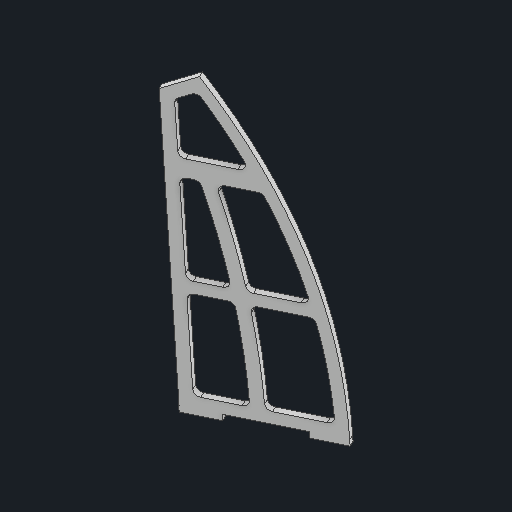
# Autodesk Inventor part: sponson_spanner_bottom
Saved by Autodesk Inventor 2023 (Build 270158030, 158C)
## iProperties
Created: 2022-03-22
Part Number: sponson_spanner_bottom
Material: Generic
Document SubType Name: Modeling
Designer: kardo
Density: 1 g/cm^3
Appearance: Default
Mass: 2.79206 g
Surface Area: 40.129 cm^2
Volume: 2.79206 cm^3
Author: kardo
Autodesk Inventor part; units mm, degrees
ref_plane "YZ Plane" through (0, 0, 0) normal (1, 0, 0) x (0, 1, 0)
ref_plane "XZ Plane" through (0, 0, 0) normal (0, 1, 0) x (-1, 0, 0)
ref_plane "XY Plane" through (0, 0, 0) normal (0, 0, 1) x (1, 0, 0)
derived "parameters_frame.ipt"
derived "stencil_frame.ipt"
sketch "sk_joint_locations" plane through (81.12, 0, 0) normal (1, 0, 0) x (0, 1, 0)
  line L0 (0, 0) -> (111.39, 7.7891) construction
  line L1 (30.81, 28.832) -> (94.8, 28.832) construction
  arc A0 (30.81, 28.832) -> (9.48, 28.5282) centre (30.81, -720.1791) ccw construction
  line L2 (-254.1001, 21.0191) -> (9.48, 28.5282) construction
  line L3 (-363, 18.496) -> (-275.8801, 20.463) construction
  arc A1 (-275.8801, 20.463) -> (-254.1001, 21.0191) centre (-359.1231, 3707.4463) ccw construction
  line L4 (-210.8824, 4616.4994) -> (225.0382, -1617.4555) construction
  line L5 (-242.0001, 4592.9714) -> (-242.0001, -1605.7041) construction
  line L6 (-120.9999, 4592.9714) -> (-120.9999, -1605.7041) construction
  line L7 (-363, 4592.9714) -> (-363, -1605.7041) construction
  line L8 (0, 4592.9714) -> (0, -1605.7041) construction
  line L9 (551.8244, 47.4419) -> (-603.6686, 7.0912) construction
  line L10 (-657.8036, -26.1228) -> (709.4042, 69.4817) construction
  line L11 (178.2183, 30.3929) -> (177.9391, 38.388) construction
  line L12 (185.9231, 36.8959) -> (186.4825, 28.8959) construction
  line L13 (0, 6.528) -> (111.1168, 11.6964) construction
  line L14 (-242.0001, 45.8501) -> (-242.0001, 21.3638) construction
  line L15 (-363, 37.4293) -> (-363, 18.496) construction
  line L16 (-120.9999, 51.0063) -> (-120.9999, 24.811) construction
  line L17 (0, 52.89) -> (0, 28.2581) construction
  line L18 (108.3896, 50.6971) -> (108.935, 42.897) construction
  line L19 (109.4805, 35.0968) -> (108.935, 42.897) construction
  line L20 (109.4805, 35.0968) -> (110.0259, 27.2967) construction
  line L21 (110.0259, 27.2967) -> (110.5713, 19.4965) construction
  line L22 (110.5713, 19.4965) -> (111.1168, 11.6964) construction
  line L23 (0, 6.528) -> (0, 0) construction
  line L24 (94.8, 37.536) -> (94.8, 28.832) construction
  line L25 (94.8, 35.548) -> (94.8, 30.82) construction
  spline S0 degree 4 poles (-363, 37.4293) (-272.3626, 45.1427) (-181.5879, 49.7528) (-90.8131, 52.89) (0, 52.89) knots 0 0 0 0 0 1 1 1 1 1
  spline S1 degree 3 poles (0, 52.89) (86.3106, 52.89) (181.3207, 49.5034) (237, 36.448) knots 0 0 0 0 1 1 1 1
  spline S2 degree 2 poles (111.39, 7.7891) (176.0348, 12.3096) (237, 36.448) knots 0 0 0 1 1 1
  point P0 (-210.8824, 4616.4994)
  point P1 (225.0382, -1617.4555)
  point P2 (178.0787, 34.3904)
  point P3 (186.2028, 32.8959)
  point P4 (134.9575, 11.3411)
  point P5 (-363, 27.9627)
  point P6 (-242.0001, 33.6069)
  point P7 (-120.9999, 37.9086)
  point P8 (0, 40.5741)
  point P9 (94.8, 33.184)
sketch "sk_spanner_joints_locations" plane through (0, 111.39, 7.7891) normal (0, 0.9975641, 0.0697565) x (-1, 0, 0)
  line L0 (270.3063, 10.9615) -> (-449.6313, 38.2305) construction
  line L1 (-853.4143, -320.9901) -> (1860.1762, 876.5297) construction
  line L2 (-85.1788, 24.4262) -> (-84.0523, 18.5329) construction
  line L3 (-85.1788, 24.4262) -> (-71.8427, 23.9211) construction
  line L4 (-84.0523, 18.5329) -> (-71.8427, 23.9211) construction
  point P0 (0, 0)
  point P1 (-126.048, 0)
  point P2 (-156, 27.1087)
  point P3 (-141.8358, 26.5722)
  point P4 (-99.343, 24.9627)
  point P5 (-94.5512, 13.8997)
  point P6 (-115.5491, 4.6332)
ref_plane "plane_strnger_outer" through (84.12, 0, 0) normal (1, 0, 0) x (0, 1, 0)
sketch "sk_corner_offset" plane through (0, 111.39, 7.7891) normal (0, 0.9975641, 0.0697565) x (-1, 0, 0)
  line L0 (-156, 27.1087) -> (-126.048, 0) construction
  line L1 (-126.048, 0) -> (-81.12, 0) construction
  point P0 (0, 0)
  point P1 (-125.5856, 1.2)
  dimension "d7" = 1.2
  dimension "d8" = 1.2
  constraints: 4 end point, 1 horizontal
  measures "d7" distance from line of L0 point (-125.586, 1.2)
  measures "d8" distance from line of point (-125.586, 1.2) L1
sketch "sk_tip_offset" plane through (81.12, 0, 0) normal (1, 0, 0) x (0, 1, 0)
  spline S0 degree 3 poles (0, 52.89) (86.3106, 52.89) (181.3207, 49.5034) (237, 36.448) knots 0 0 0 0 1 1 1 1 construction
  spline S1 degree 2 poles (111.39, 7.7891) (176.0348, 12.3096) (237, 36.448) knots 0 0 0 1 1 1 construction
  spline S2 degree 5 poles (0, 51.69) (13.1181, 51.69) (26.2363, 51.6248) (39.354, 51.4874) (65.3463, 51.0551) (91.3298, 50.254) (104.1978, 49.754) (128.8047, 48.5691) (153.3792, 46.8416) (165.0971, 45.8705) (185.7675, 43.844) (206.3487, 41.0607) (215.2522, 39.6762) (224.1241, 38.0772) (232.9228, 36.143) knots 0 0 0 0 0 0 0.280538 0.280538 0.280538 0.555921 0.555921 0.555921 0.807344 0.807344 0.807344 1 1 1 1 1 1
  spline S3 degree 5 poles (111.3063, 8.9862) (136.261, 10.7315) (161.0871, 14.3225) (185.5959, 19.817) (209.5823, 27.1424) (232.9228, 36.1431) knots 0 0 0 0 0 0 1 1 1 1 1 1
  point P0 (0, 0)
  dimension "d9" = 1.2
  dimension "d10" = 1.2
  constraints: 1 coincident, 6 other
sketch "sk_spanner_bottom_base" plane through (126.048, 0, 0) normal (0.4037383, -0.0638184, 0.9126459) x (-0.1841621, 0.9714748, 0.1494022)
  spline S0 degree 2 poles (109.3763, -22.4773) (178.4423, -36.6707) (243.959, 0) knots 0 0 0 1 1 1 construction
  line L0 (-581.1403, 166.2138) -> (698.1316, -96.6821) projected
  line L1 (109.559, -21.5883) -> (107.5999, -21.1858)
  line L2 (107.5999, -21.1858) -> (109.7273, -10.8338)
  line L3 (109.7273, -10.8338) -> (111.6863, -11.2364)
  line L4 (111.6863, -11.2364) -> (116.3065, 11.2454)
  line L5 (116.3065, 11.2454) -> (114.3474, 11.648)
  line L6 (114.3474, 11.648) -> (116.6574, 22.8889)
  line L7 (116.6574, 22.8889) -> (118.6165, 22.4863)
  line L8 (118.6165, 22.4863) -> (118.6016, 22.4138)
  line L9 (109.3763, -22.4773) -> (0, 0) construction
  spline S1 degree 2 poles (109.559, -21.5883) (176.5828, -35.362) (239.9525, 0.8152) knots 0 0 0 1 1 1
  point P0 (23.2133, 112.9576)
  point P1 (194.0801, 10.2503)
  point P2 (239.5045, -2.4323)
  point P3 (0, 0)
  point P4 (235.5713, -1.624)
  dimension "d4" = 2
  constraints: 16 end point, 3 parallel, 2 collinear, 2 perpendicular, 1 point on line, 5 other
  measures "d4" distance between parallel lines of L6 L4
extrude "thicken" add sketch "sk_spanner_bottom_base" along normal blind 2
sketch "sk_cut_weight" plane through (126.048, 0, 0) normal (0.4037383, -0.0638184, 0.9126459) x (-0.1841621, 0.9714748, 0.1494022)
  spline S0 degree 2 poles (109.559, -21.5883) (176.5828, -35.362) (239.9525, 0.8152) knots 0 0 0 1 1 1 construction
  line L0 (-581.1403, 166.2138) -> (698.1316, -96.6821) projected
  line L1 (111.6863, -11.2364) -> (116.3065, 11.2454) construction
  line L2 (118.6165, 22.4863) -> (118.6016, 22.4138) projected
  line L3 (194.0801, 10.2503) -> (187.7911, -20.3522) construction
  line L4 (118.6165, 22.4863) -> (189.5168, 7.916)
  line L5 (189.5168, 7.916) -> (189.5019, 7.8435)
  line L6 (195.379, 6.6357) -> (195.3939, 6.7082)
  line L7 (195.3939, 6.7082) -> (235.5862, -1.5515)
  line L8 (121.7294, 17.763) -> (188.7116, 3.9979)
  line L9 (188.7116, 3.9979) -> (187.6316, -1.2574)
  line L10 (121.7294, 17.763) -> (118.7255, 3.1454)
  line L11 (194.5887, 2.7901) -> (190.7538, -15.8709)
  line L12 (235.5862, -1.5515) -> (235.5713, -1.624)
  spline S1 degree 2 poles (113.9964, 0.0045) (151.9369, -7.7924) (190.9356, -5.0509) knots 0 0 0 1 1 1
  line L13 (194.5887, 2.7901) -> (224.3355, -3.323)
  line L14 (186.7983, -5.3123) -> (184.2993, -17.4727)
  line L15 (117.9202, -0.7731) -> (114.2114, -18.8203)
  line L16 (157.1796, 10.4778) -> (154.7576, -1.3076)
  line L17 (153.2614, 11.283) -> (150.7276, -1.0469)
  line L18 (153.944, -5.2669) -> (150.5615, -21.726)
  line L19 (149.9156, -4.9983) -> (146.4667, -21.7805)
  line L20 (155.2205, 10.8804) -> (148.5116, -21.7656) construction
  line L21 (215.49, 2.5784) -> (228.4331, -36.359)
  line L22 (212.4227, -0.8749) -> (214.6796, -7.6643)
  line L23 (235.5862, -1.5515) -> (228.4331, -36.359)
  spline S2 degree 5 poles (114.2114, -18.8202) (126.2441, -21.0287) (138.4561, -22.2563) (150.7607, -22.3923) (173.4033, -20.5426) (195.4165, -15.0261) (205.3202, -11.7541) (214.9665, -7.8266) (224.3355, -3.323) knots 0 0 0 0 0 0 0.540618 0.540618 0.540618 1 1 1 1 1 1
  spline S3 degree 4 poles (114.8016, 3.9226) (123.6889, 2.0961) (132.6562, 0.6525) (141.6777, -0.395) (150.7276, -1.0469) knots 0 0 0 0 0 1 1 1 1 1
  spline S4 degree 4 poles (150.7276, -1.0469) (159.9364, -1.7102) (169.1747, -1.9637) (178.4154, -1.8078) (187.6316, -1.2573) knots 0 0 0 0 0 1 1 1 1 1
  point P0 (23.2133, 112.9576)
  point P1 (154.7576, -1.3076)
  dimension "d11" = 3.6057
  dimension "d17" = 4
  dimension "d12" = 2
  dimension "d13" = 4
  dimension "d14" = 4
  dimension "d15" = 4
  dimension "d18" = 4
  dimension "d22" = 60
  dimension "d23" = 4
  constraints: 43 end point, 9 collinear, 7 point on line, 6 parallel, 5 perpendicular, 4 midpoint, 29 other
  measures "d12" distance between parallel lines of L6 L3
  measures "d13" distance between parallel lines of L3 L5
  measures "d14" distance between parallel lines of L4 L8
  measures "d15" distance between parallel lines of L1 L10
  measures "d18" distance between parallel lines of L17 L16
  measures "d22" angle of L7 L21
  measures "d23" distance between parallel lines of L22 L21
extrude "cut_weight" cut sketch "sk_cut_weight" along normal through all both and the other way through all contours L2 L4 L5 L0 | L6 L7 L21 L0 | L21 L7 L12 L0 | L0 L23 L21 S2 L13 | L13 S2 L21 | L22 S2 L11 L13 | L8 L17 S3 L10 | L8 L9 S4 L16 | S1 L19 S2 L15 | S1 L14 S2 L18
fillet "rounding" radius 2 20 edges at (88.1155, 188.337, 31.0462) (88.1155, 150.2391, 28.3821) (102.821, 150.6918, 21.9083) (105.4282, 114.6693, 18.236) (88.1155, 114.1363, 25.8575) (88.1155, 146.2488, 28.1031) (103.3221, 146.717, 21.4087) (88.1155, 182.3516, 30.6276) (96.8112, 182.6193, 26.7996) (93.0239, 182.5027, 28.4668) (108.1689, 182.9689, 21.7996) (118.9967, 147.1995, 14.5083) (99.6316, 146.6033, 23.0334) (105.5447, 188.8735, 23.3733) (118.1937, 151.165, 15.1408) (122.2841, 115.1881, 10.8155) (99.1231, 150.5779, 23.5363) (101.7683, 114.5566, 19.8472) (88.1155, 206.4993, 32.3162) (93.7843, 210.2425, 30.0702)
equation "\"d7\" = shell_thickness"
equation "\"d8\" = shell_thickness"
equation "\"d9\" = shell_thickness"
equation "\"d10\" = shell_thickness"
equation "\"d4\" = bulkhead_thickness"
equation "\"d5\" = bulkhead_thickness"
equation "\"d17\" = bulkhead_inset"
equation "\"d12\" = bulkhead_thickness"
equation "\"d13\" = 2 * bulkhead_thickness"
equation "\"d14\" = bulkhead_inset"
equation "\"d15\" = bulkhead_inset"
equation "\"d18\" = bulkhead_inset"
equation "\"d23\" = bulkhead_inset"
equation "\"d21\" = 0.5 * bulkhead_inset"
equation "\"d3\" = stringer_thickness"
equation "\"shell_thickness\" = 1.2"
equation "\"bulkhead_thickness\" = 2"
equation "\"bulkhead_inset\" = 4"
equation "\"stringer_thickness\" = 3"
body "Solid1"
